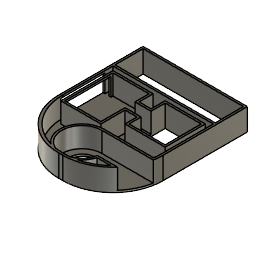
[vacc]base2 (Autodesk Fusion 360 design; units mm, degrees)
part number: 2026-07-20-20-28-10-473
Autodesk Fusion 360 part; units mm, degrees
sketch "Sketch1" plane through (0, 0, 0) normal (0, 0, 1) x (1, 0, 0)
  line L0 (-25, 25) -> (235, 25)
  line L1 (235, 25) -> (235, -110)
  line L2 (110, -235) -> (100, -235)
  line L3 (-25, -110) -> (-25, 25)
  line L4 (-25, 25) -> (-20, 25)
  line L5 (-20, 25) -> (-20, 20)
  line L6 (-20, 20) -> (-25, 20)
  line L7 (-25, 20) -> (-25, 25)
  line L8 (235, 25) -> (230, 25)
  line L9 (230, 25) -> (230, 20)
  line L10 (230, 20) -> (235, 20)
  line L11 (235, 20) -> (235, 25)
  line L12 (-25, -235) -> (-20, -235)
  line L13 (-20, -235) -> (-20, -230)
  line L14 (-20, -230) -> (-25, -230)
  line L15 (-25, -230) -> (-25, -235)
  line L16 (235, -235) -> (230, -235)
  line L17 (230, -235) -> (230, -230)
  line L18 (230, -230) -> (235, -230)
  line L19 (235, -230) -> (235, -235)
  line L20 (-20, 20) -> (230, 20)
  line L21 (230, 20) -> (230, -110)
  line L22 (110, -230) -> (100, -230)
  line L23 (-20, -110) -> (-20, 20)
  arc A0 (-20, -110) -> (100, -230) centre (100, -110) ccw
  arc A1 (-25, -110) -> (100, -235) centre (100, -110) ccw
  arc A2 (110, -230) -> (230, -110) centre (110, -110) ccw
  arc A3 (110, -235) -> (235, -110) centre (110, -110) ccw
  dimension "d1" = 260
  dimension "d2" = 260
  dimension "d3" = 5
  dimension "d4" = 5
  dimension "d5" = 120
  dimension "d6" = 125
  dimension "d7" = 120
  dimension "d8" = 125
  constraint horizontal L0
  constraint vertical L1
  constraint horizontal L2
  constraint vertical L3
  constraint horizontal L4
  constraint vertical L5
  constraint horizontal L6
  constraint vertical L7
  constraint horizontal L8
  constraint vertical L9
  constraint horizontal L10
  constraint vertical L11
  constraint horizontal L12
  constraint vertical L13
  constraint horizontal L14
  constraint vertical L15
  constraint horizontal L16
  constraint vertical L17
  constraint horizontal L18
  constraint vertical L19
  constraint horizontal L20
  constraint vertical L21
  constraint horizontal L22
  constraint vertical L23
  constraint tangent L23 A0
  constraint tangent L22 A0
  constraint coincident L12.start L3
  constraint coincident L12.start L2
  constraint tangent L3 A1
  constraint tangent L2 A1
  constraint coincident L17.end L21
  constraint coincident L17.end L22
  constraint tangent L21 A2
  constraint tangent L22 A2
  constraint coincident L16.start L2
  constraint coincident L16.start L1
  constraint tangent L2 A3
  constraint tangent L1 A3
  measures "d1" distance of L0.start L12.start
  measures "d2" distance of L0.start L0.end
  measures "d3" distance of L0.start L4.end
  measures "d4" distance of L0.start L6.end
  measures "d5" radius of A0
  measures "d6" radius of A1
  measures "d7" radius of A2
  measures "d8" radius of A3
extrude "Extrude1" add sketch "Sketch1" along normal blind 5 contours L0 L3 L4 L5 L6 L7 | L0 L5 L9 L20 | L1 L2 L3 L6 L10 L21 L22 L23 A0 A1 A2 A3 | L0 L1 L8 L9 L10 L11 | L20 L21 L22 L23 A0 A2
sketch "Sketch2" plane through (0, 0, 5) normal (0, 0, 1) x (-1, 0, 0)
  arc A0 (25, 110) -> (-100, 235) centre (-100, 110) ccw
  line L0 (-100, 235) -> (-110, 235)
  arc A1 (-110, 235) -> (-235, 110) centre (-110, 110) ccw
  line L1 (-235, 110) -> (-235, -25)
  line L2 (-235, -25) -> (25, -25)
  line L3 (25, -25) -> (25, 110)
  line L4 (25, -25) -> (-235, -25)
  line L5 (-235, -25) -> (-235, 110)
  line L6 (-110, 235) -> (-100, 235)
  line L7 (25, 110) -> (25, -25)
  line L8 (25, -25) -> (20, -25)
  line L9 (20, -25) -> (20, -20)
  line L10 (20, -20) -> (25, -20)
  line L11 (25, -20) -> (25, -25)
  line L12 (-235, -25) -> (-230, -25)
  line L13 (-230, -25) -> (-230, -20)
  line L14 (-230, -20) -> (-235, -20)
  line L15 (-235, -20) -> (-235, -25)
  line L16 (25, 235) -> (20, 235)
  line L17 (20, 235) -> (20, 230)
  line L18 (20, 230) -> (25, 230)
  line L19 (25, 230) -> (25, 235)
  line L20 (-235, 235) -> (-230, 235)
  line L21 (-230, 235) -> (-230, 230)
  line L22 (-230, 230) -> (-235, 230)
  line L23 (-235, 230) -> (-235, 235)
  line L24 (20, -20) -> (-230, -20)
  line L25 (-230, -20) -> (-230, 110)
  line L26 (-110, 230) -> (-105, 230)
  line L27 (20, 105) -> (20, -20)
  arc A2 (20, 105) -> (-105, 230) centre (-105, 105) ccw
  arc A3 (25, 110) -> (-100, 235) centre (-100, 110) ccw
  arc A4 (-110, 230) -> (-230, 110) centre (-110, 110) ccw
  arc A5 (-110, 235) -> (-235, 110) centre (-110, 110) ccw
  dimension "d11" = 260
  dimension "d12" = 260
  dimension "d13" = 5
  dimension "d14" = 5
  dimension "d15" = 5
  dimension "d16" = 5
  dimension "d17" = 125
  dimension "d18" = 120
  dimension "d19" = 125
  constraint horizontal L4
  constraint vertical L5
  constraint horizontal L6
  constraint vertical L7
  constraint coincident L2.end L3.start
  constraint horizontal L8
  constraint vertical L9
  constraint horizontal L10
  constraint vertical L11
  constraint horizontal L12
  constraint vertical L13
  constraint horizontal L14
  constraint vertical L15
  constraint coincident L1.end L2.start
  constraint horizontal L16
  constraint vertical L17
  constraint horizontal L18
  constraint vertical L19
  constraint horizontal L20
  constraint vertical L21
  constraint horizontal L22
  constraint vertical L23
  constraint horizontal L24
  constraint vertical L25
  constraint horizontal L26
  constraint vertical L27
  constraint tangent L27 A2
  constraint tangent L26 A2
  constraint coincident L16.start L7
  constraint coincident L16.start L6
  constraint tangent L7 A3
  constraint tangent L6 A3
  constraint equal A2 A3
  constraint coincident L21.end L25
  constraint coincident L21.end L26
  constraint tangent L25 A4
  constraint tangent L26 A4
  constraint coincident L20.start L6
  constraint coincident L20.start L5
  constraint tangent L6 A5
  constraint tangent L5 A5
  measures "d11" distance of L2.end L16.start
  measures "d12" distance of L20.start L16.start
  measures "d13" distance of L17.end L18.end
  measures "d14" distance of L16.end L17.end
  measures "d15" distance of L21.end L22.end
  measures "d16" distance of L20.end L21.end
  measures "d17" radius of A2
  measures "d18" radius of A4
  measures "d19" radius of A5
extrude "Extrude2" add sketch "Sketch2" along normal blind 50 contours A0 L0 A1 L1 L3 L5 L6 L7 L10 L14 L25 L26 L27 A2 A3 A4 A5 | L2 L3 L4 L7 L8 L9 L10 L11 | L2 L4 L9 L13 L24 | L1 L2 L4 L5 L12 L13 L14 L15
sketch "Sketch3" plane through (0, 0, 5) normal (0, 0, 1) x (-1, 0, 0)
  line L0 (-105, 230) -> (-110, 230)
  arc A0 (-110, 230) -> (-230, 110) centre (-110, 110) ccw
  line L1 (-230, 110) -> (-230, -20)
  line L2 (-230, -20) -> (20, -20)
  line L3 (20, -20) -> (20, 105)
  arc A1 (20, 105) -> (-105, 230) centre (-105, 105) ccw
  line L4 (-230, -20) -> (-220, -20)
  line L5 (-220, -20) -> (-220, -10)
  line L6 (-220, -10) -> (-120, -10)
  line L7 (-120, -10) -> (-120, 90)
  line L8 (-120, 90) -> (-220, 90)
  line L9 (-220, 90) -> (-220, -10)
  line L10 (20, -20) -> (20, -10)
  line L11 (20, -20) -> (10, -20)
  line L12 (20, -20) -> (10, -20)
  line L13 (10, -20) -> (10, -10)
  line L14 (10, -10) -> (20, -10)
  line L15 (20, -10) -> (20, -20)
  line L16 (10, -10) -> (-90, -10)
  line L17 (-90, -10) -> (-90, 120)
  line L18 (-90, 120) -> (10, 120)
  line L19 (10, 120) -> (10, -10)
  line L20 (-90, -10) -> (-90, 30)
  line L21 (-120, -10) -> (-120, 30)
  line L22 (-120, 30) -> (-90, 30)
  line L23 (-90, 30) -> (-90, 55)
  line L24 (-90, 55) -> (-120, 55)
  line L25 (-120, 55) -> (-120, 30)
  line L26 (10, -10) -> (5, -10)
  line L27 (5, -10) -> (5, -5)
  line L28 (5, -5) -> (10, -5)
  line L29 (10, -5) -> (10, -10)
  line L30 (-90, -10) -> (-85, -10)
  line L31 (-85, -10) -> (-85, -5)
  line L32 (-85, -5) -> (-90, -5)
  line L33 (-90, -5) -> (-90, -10)
  line L34 (10, 120) -> (5, 120)
  line L35 (5, 120) -> (5, 115)
  line L36 (5, 115) -> (10, 115)
  line L37 (10, 115) -> (10, 120)
  line L38 (-90, 120) -> (-85, 120)
  line L39 (-85, 120) -> (-85, 115)
  line L40 (-85, 115) -> (-90, 115)
  line L41 (-90, 115) -> (-90, 120)
  line L42 (5, -5) -> (-85, -5)
  line L43 (-85, -5) -> (-85, 115)
  line L44 (-85, 115) -> (5, 115)
  line L45 (5, 115) -> (5, -5)
  line L46 (-90, 30) -> (-90, 25)
  line L47 (-120, 30) -> (-120, 25)
  line L48 (-120, 25) -> (-90, 25)
  line L49 (-90, 55) -> (-90, 60)
  line L50 (-120, 55) -> (-120, 60)
  line L51 (-120, 60) -> (-90, 60)
  line L52 (-120, -10) -> (-125, -10)
  line L53 (-125, -10) -> (-125, -5)
  line L54 (-125, -5) -> (-120, -5)
  line L55 (-120, -5) -> (-120, -10)
  line L56 (-220, -10) -> (-215, -10)
  line L57 (-215, -10) -> (-215, -5)
  line L58 (-215, -5) -> (-220, -5)
  line L59 (-220, -5) -> (-220, -10)
  line L60 (-120, 90) -> (-125, 90)
  line L61 (-125, 90) -> (-125, 85)
  line L62 (-125, 85) -> (-120, 85)
  line L63 (-120, 85) -> (-120, 90)
  line L64 (-220, 90) -> (-215, 90)
  line L65 (-215, 90) -> (-215, 85)
  line L66 (-215, 85) -> (-220, 85)
  line L67 (-220, 85) -> (-220, 90)
  line L68 (-125, -5) -> (-215, -5)
  line L69 (-215, -5) -> (-215, 85)
  line L70 (-215, 85) -> (-125, 85)
  line L71 (-125, 85) -> (-125, -5)
  dimension "d22" = 10
  dimension "d23" = 10
  dimension "d24" = 100
  dimension "d25" = 100
  dimension "d26" = 10
  dimension "d27" = 10
  dimension "d28" = 100
  dimension "d29" = 130
  dimension "d30" = 40
  dimension "d31" = 30
  dimension "d32" = 25
  dimension "d33" = 5
  dimension "d34" = 5
  constraint coincident L1.end L2.start
  constraint perpendicular L1 L4
  constraint perpendicular L4 L5
  constraint horizontal L6
  constraint vertical L7
  constraint horizontal L8
  constraint vertical L9
  constraint coincident L2.end L3.start
  constraint perpendicular L2 L10
  constraint coincident L2 L11.end
  constraint horizontal L12
  constraint vertical L13
  constraint horizontal L14
  constraint vertical L15
  constraint horizontal L16
  constraint vertical L17
  constraint horizontal L18
  constraint vertical L19
  constraint coincident L17 L20.end
  constraint perpendicular L16 L21
  constraint horizontal L22
  constraint vertical L23
  constraint horizontal L24
  constraint vertical L25
  constraint midpoint L17 L23.end
  constraint horizontal L26
  constraint vertical L27
  constraint horizontal L28
  constraint vertical L29
  constraint horizontal L30
  constraint vertical L31
  constraint horizontal L32
  constraint vertical L33
  constraint horizontal L34
  constraint vertical L35
  constraint horizontal L36
  constraint vertical L37
  constraint horizontal L38
  constraint vertical L39
  constraint horizontal L40
  constraint vertical L41
  constraint horizontal L42
  constraint vertical L43
  constraint horizontal L44
  constraint vertical L45
  constraint coincident L17 L46.end
  constraint coincident L21 L47.end
  constraint perpendicular L46 L48
  constraint coincident L17 L49.end
  constraint coincident L7 L50.end
  constraint perpendicular L49 L51
  constraint horizontal L52
  constraint vertical L53
  constraint horizontal L54
  constraint vertical L55
  constraint horizontal L56
  constraint vertical L57
  constraint horizontal L58
  constraint vertical L59
  constraint horizontal L60
  constraint vertical L61
  constraint horizontal L62
  constraint vertical L63
  constraint horizontal L64
  constraint vertical L65
  constraint horizontal L66
  constraint vertical L67
  constraint horizontal L68
  constraint vertical L69
  constraint horizontal L70
  constraint vertical L71
  measures "d22" distance of L1.end L4.end
  measures "d23" distance of L4.end L5.end
  measures "d24" distance of L5.end L6.end
  measures "d25" distance of L5.end L8.end
  measures "d26" distance of L1 L8.end
  measures "d27" distance of L2.end L10.end
  measures "d28" distance of L13.end L16.end
  measures "d29" distance of L13.end L18.end
  measures "d30" distance of L6.end L21.end
  measures "d31" distance of L21.end L20.end
  measures "d32" distance of L20.end L23.end
  measures "d33" distance of L21.end L47.end
  measures "d34" distance of L24.end L50.end
extrude "Extrude3" add sketch "Sketch3" along normal blind 50 contours L16 L19 L26 L27 L28 L29 | L16 L27 L31 L42 | L19 L28 L36 L45 | L6 L9 L56 L57 L58 L59 | L16 L17 L20 L30 L31 L32 L33 | L18 L19 L34 L35 L36 L37 | L6 L53 L57 L68 | L9 L58 L66 L69 | L17 L20 L23 L32 L40 L43 L46 L49 | L18 L35 L39 L44 | L6 L7 L21 L52 L53 L54 L55 | L8 L9 L64 L65 L66 L67 | L17 L18 L38 L39 L40 L41 | L7 L21 L25 L47 L50 L54 L62 L71 | L8 L61 L65 L70 | L7 L17 L20 L21 L22 L46 L47 L48 | L7 L8 L60 L61 L62 L63 | L7 L17 L24 L49 L50 L51
extrude "Extrude4" cut 1 faces at (90, -38.3333, 21.6667) along direction (-1, 0, 0) blind 20
extrude "Extrude5" cut 1 faces at (120, -38.3333, 21.6667) along direction (1, 0, 0) blind 30
sketch "Sketch4" plane through (0, 0, 5) normal (0, 0, 1) x (-1, 0, 0)
  line L0 (-85, 55) -> (-125, 55)
  line L1 (-125, 55) -> (-125, 85)
  line L2 (-125, 85) -> (-215, 85)
  line L3 (-215, 85) -> (-215, -5)
  line L4 (-215, -5) -> (-125, -5)
  line L5 (-125, -5) -> (-125, 30)
  line L6 (-125, 30) -> (-85, 30)
  line L7 (-85, 30) -> (-85, -5)
  line L8 (-85, -5) -> (5, -5)
  line L9 (5, -5) -> (5, 115)
  line L10 (5, 115) -> (-85, 115)
  line L11 (-85, 115) -> (-85, 55)
  line L12 (-125, -5) -> (-215, -5)
  line L13 (-215, -5) -> (-215, 85)
  line L14 (-215, 85) -> (-125, 85)
  line L15 (-125, 85) -> (-125, -5)
  constraint horizontal L12
  constraint vertical L13
  constraint horizontal L14
  constraint vertical L15
  constraint coincident L2.end L3.start
  constraint coincident L4.end L5.start
extrude "Extrude6" cut sketch "Sketch4" against normal blind 30 contours L1 L2 L3 L4 L5 L12 L13 L14 L15
sketch "Sketch5" plane through (0, 0, 5) normal (0, 0, 1) x (-1, 0, 0)
  line L0 (-105, 230) -> (-110, 230)
  arc A0 (-110, 230) -> (-230, 110) centre (-110, 110) ccw
  line L1 (-230, 110) -> (-230, -20)
  line L2 (-230, -20) -> (20, -20)
  line L3 (20, -20) -> (20, 105)
  arc A1 (20, 105) -> (-105, 230) centre (-105, 105) ccw
  line L4 (-220, 90) -> (-120, 90)
  line L5 (-120, 90) -> (-120, 60)
  line L6 (-120, 60) -> (-90, 60)
  line L7 (-90, 60) -> (-90, 120)
  line L8 (-90, 120) -> (10, 120)
  line L9 (10, 120) -> (10, -10)
  line L10 (10, -10) -> (-90, -10)
  line L11 (-90, -10) -> (-90, 25)
  line L12 (-90, 25) -> (-120, 25)
  line L13 (-120, 25) -> (-120, -10)
  line L14 (-120, -10) -> (-220, -10)
  line L15 (-220, -10) -> (-220, 90)
  line L16 (25, -25) -> (-235, -25)
  line L17 (-235, -25) -> (-235, 235)
  line L18 (-235, 235) -> (25, 235)
  line L19 (25, 235) -> (25, -25)
  line L20 (25, -25) -> (20, -25)
  line L21 (20, -25) -> (20, -20)
  line L22 (20, -20) -> (25, -20)
  line L23 (25, -20) -> (25, -25)
  line L24 (-235, -25) -> (-230, -25)
  line L25 (-230, -25) -> (-230, -20)
  line L26 (-230, -20) -> (-235, -20)
  line L27 (-235, -20) -> (-235, -25)
  line L28 (25, 235) -> (20, 235)
  line L29 (20, 235) -> (20, 230)
  line L30 (20, 230) -> (25, 230)
  line L31 (25, 230) -> (25, 235)
  line L32 (-235, 235) -> (-230, 235)
  line L33 (-230, 235) -> (-230, 232.5)
  line L34 (-230, 232.5) -> (-235, 232.5)
  line L35 (-235, 232.5) -> (-235, 235)
  line L36 (20, -20) -> (-230, -20)
  line L37 (-230, -20) -> (-230, 232.5)
  line L38 (-230, 232.5) -> (20, 232.5)
  line L39 (20, 232.5) -> (20, -20)
  line L40 (20, 232.5) -> (20, 182.5)
  line L41 (-230, 232.5) -> (-230, 182.5)
  line L42 (20, 182.5) -> (-105, 182.5)
  circle A2 centre (-105, 182.5) radius 50
  line L43 (-55, 182.5) -> (-155, 182.5)
  line L44 (-155, 182.5) -> (-155, 235)
  line L45 (-155, 235) -> (-55, 235)
  line L46 (-55, 235) -> (-55, 182.5)
  line L47 (-230, 182.5) -> (-230, 142.5)
  line L48 (-105, 182.5) -> (-105, 132.5)
  line L49 (-105, 132.5) -> (-235, 132.5)
  line L50 (-230, 132.5) -> (-230, 182.5)
  line L51 (-230, 182.5) -> (-230, 192.5)
  line L52 (-230, 192.5) -> (-153.9898, 192.5)
  circle A3 centre (-105, 182.5) radius 55
  line L53 (-105, 127.5) -> (-235, 127.5)
  line L54 (-230, 192.5) -> (-230, 197.5)
  line L55 (-230, 132.5) -> (-230, 192.5)
  line L56 (20, 182.5) -> (-160, 182.5)
  line L57 (-230, 197.5) -> (-157.915, 197.5)
  dimension "d43" = 260
  dimension "d44" = 260
  dimension "d45" = 5
  dimension "d46" = 5
  dimension "d47" = 50
  dimension "d48" = 50
  dimension "d49" = 125
  dimension "d50" = 100
  dimension "d51" = 40
  dimension "d52" = 50
  dimension "d53" = 10
  dimension "d54" = 110
  dimension "d55" = 5
  dimension "d56" = 5
  dimension "d57" = 60
  constraint horizontal L16
  constraint vertical L17
  constraint horizontal L18
  constraint vertical L19
  constraint horizontal L20
  constraint vertical L21
  constraint horizontal L22
  constraint vertical L23
  constraint coincident L2.end L3.start
  constraint horizontal L24
  constraint vertical L25
  constraint horizontal L26
  constraint vertical L27
  constraint coincident L1.end L2.start
  constraint horizontal L28
  constraint vertical L29
  constraint horizontal L30
  constraint vertical L31
  constraint horizontal L32
  constraint vertical L33
  constraint horizontal L34
  constraint vertical L35
  constraint horizontal L36
  constraint vertical L37
  constraint horizontal L38
  constraint vertical L39
  constraint perpendicular L38 L40
  constraint perpendicular L38 L41
  constraint coincident L42.end A2.centre
  constraint horizontal L43
  constraint vertical L44
  constraint horizontal L45
  constraint vertical L46
  constraint coincident L18 L44.end
  constraint coincident A2 L43.start
  constraint coincident L43.start L56
  constraint coincident A2 L48.end
  constraint perpendicular L42 L48
  constraint coincident L17 L49.end
  constraint perpendicular L17 L49
  constraint coincident L49 L50.start
  constraint coincident L37 L50.start
  constraint coincident A2 L52.end
  constraint perpendicular L44 L52
  constraint concentric A2 A3
  constraint coincident A3 L53.start
  constraint coincident L17 L53.end
  constraint tangent A3 L53
  constraint perpendicular L17 L53
  constraint perpendicular L52 L54
  constraint parallel L41 L55
  constraint coincident A3 L56.end
  constraint coincident L42.end L56
  constraint coincident A3 L57.end
  constraint perpendicular L54 L57
  measures "d43" distance of L16.start L16.end
  measures "d44" distance of L16.start L18.end
  measures "d45" distance of L29.end L30.end
  measures "d46" distance of L28.end L29.end
  measures "d47" distance of L38.end L40.end
  measures "d48" distance of L33.end L41.end
  measures "d49" distance of L40.end L42.end
  measures "d50" diameter of A2
  measures "d51" distance of L41.end L47.end
  measures "d52" distance of L41.end L50.start
  measures "d53" distance of L41.end L51.end
  measures "d54" diameter of A3
  measures "d55" distance of L51.end L54.end
  measures "d56" distance of L49 L53
  measures "d57" distance of L50.start L51.end
extrude "Extrude7" add sketch "Sketch5" along normal blind 50 contours A1 A2 L46 A3 | A0 A2 L44 L52 A3 | L42 L46 A3 L56 | L42 A2 L49 A3 L56 | L44 L52 A3 | A0 L49 A3 L53 | A0 L52 A3 L57
sketch "Sketch6" plane through (0, 0, 5) normal (0, 0, 1) x (-1, 0, 0)
  line L0 (-227.8718, 132.5) -> (-105, 132.5)
  arc A0 (-105, 132.5) -> (-85.2346, 228.4274) centre (-105, 182.5) ccw
  arc A1 (-85.2346, 228.4274) -> (-105, 230) centre (-105, 105) ccw
  line L1 (-105, 230) -> (-110, 230)
  arc A2 (-110, 230) -> (-122.4639, 229.351) centre (-110, 110) ccw
  arc A3 (-122.4639, 229.351) -> (-153.9898, 192.5) centre (-105, 182.5) ccw
  line L2 (-153.9898, 192.5) -> (-197.1421, 192.5)
  arc A4 (-197.1421, 192.5) -> (-227.8718, 132.5) centre (-110, 110) ccw
  line L3 (25.0024, -24.9997) -> (-234.9976, -24.9997)
  line L4 (-234.9976, -24.9997) -> (-234.9976, 235.0003)
  line L5 (-234.9976, 235.0003) -> (25.0024, 235.0003)
  line L6 (25.0024, 235.0003) -> (25.0024, -24.9997)
  line L7 (25.0024, -24.9997) -> (20.0024, -24.9997)
  line L8 (20.0024, -24.9997) -> (20.0024, -19.9997)
  line L9 (20.0024, -19.9997) -> (25.0024, -19.9997)
  line L10 (25.0024, -19.9997) -> (25.0024, -24.9997)
  line L11 (-234.9976, -24.9997) -> (-229.9976, -24.9997)
  line L12 (-229.9976, -24.9997) -> (-229.9976, -20)
  line L13 (-229.9976, -20) -> (-234.9976, -20)
  line L14 (-234.9976, -20) -> (-234.9976, -24.9997)
  line L15 (25.0024, 235.0003) -> (20.0024, 235.0003)
  line L16 (20.0024, 235.0003) -> (20.0024, 230)
  line L17 (20.0024, 230) -> (25.0024, 230)
  line L18 (25.0024, 230) -> (25.0024, 235.0003)
  line L19 (-234.9976, 235.0003) -> (-229.9976, 235.0003)
  line L20 (-229.9976, 235.0003) -> (-229.9976, 230)
  line L21 (-229.9976, 230) -> (-234.9976, 230)
  line L22 (-234.9976, 230) -> (-234.9976, 235.0003)
  line L23 (20.0024, -19.9997) -> (-229.9976, -19.9997)
  line L24 (-229.9976, -19.9997) -> (-229.9976, 230)
  line L25 (-229.9976, 230) -> (20.0024, 230)
  line L26 (20.0024, 230) -> (20.0024, -19.9997)
  line L27 (20.0024, 230) -> (20.0024, 180)
  line L28 (-229.9976, 230) -> (-229.9976, 180)
  line L29 (20.0024, 180) -> (-229.9976, 180)
  line L30 (20.0024, 180) -> (-104.9976, 180)
  circle A5 centre (-104.9976, 180) radius 32
  dimension "d60" = 260
  dimension "d61" = 260
  dimension "d62" = 5
  dimension "d63" = 5
  dimension "d64" = 5
  dimension "d65" = 5
  dimension "d66" = 5
  dimension "d67" = 50
  dimension "d68" = 50
  dimension "d69" = 125
  dimension "d70" = 64
  constraint horizontal L3
  constraint vertical L4
  constraint horizontal L5
  constraint vertical L6
  constraint horizontal L7
  constraint vertical L8
  constraint horizontal L9
  constraint vertical L10
  constraint horizontal L11
  constraint vertical L12
  constraint horizontal L13
  constraint vertical L14
  constraint horizontal L15
  constraint vertical L16
  constraint horizontal L17
  constraint vertical L18
  constraint horizontal L19
  constraint vertical L20
  constraint horizontal L21
  constraint vertical L22
  constraint horizontal L23
  constraint vertical L24
  constraint horizontal L25
  constraint vertical L26
  constraint perpendicular L17 L27
  constraint perpendicular L25 L28
  constraint perpendicular L24 L29
  constraint midpoint L29 L30.end
  constraint coincident L30.end A5.centre
  measures "d60" distance of L3.start L5.end
  measures "d61" distance of L4.end L5.end
  measures "d62" distance of L3.start L9.end
  measures "d63" distance of L3.start L7.end
  measures "d64" distance of L3.end L11.end
  measures "d65" distance of L5.end L15.end
  measures "d66" distance of L4.end L19.end
  measures "d67" distance of L16.end L27.end
  measures "d68" distance of L20.end L28.end
  measures "d69" distance of L27.end L30.end
  measures "d70" diameter of A5
extrude "Extrude8" cut sketch "Sketch6" against normal blind 30 contours L29 L30 A5 | L29 L30 A5
sketch "Sketch7" plane through (0, 0, 5) normal (0, 0, 1) x (-1, 0, 0)
  circle A0 centre (-104.9976, 180) radius 32
  line L0 (-227.8718, 132.5) -> (-105, 132.5)
  arc A1 (-105, 132.5) -> (-85.2346, 228.4274) centre (-105, 182.5) ccw
  arc A2 (-85.2346, 228.4274) -> (-105, 230) centre (-105, 105) ccw
  line L1 (-105, 230) -> (-110, 230)
  arc A3 (-110, 230) -> (-122.4639, 229.351) centre (-110, 110) ccw
  arc A4 (-122.4639, 229.351) -> (-153.9898, 192.5) centre (-105, 182.5) ccw
  line L2 (-153.9898, 192.5) -> (-197.1421, 192.5)
  arc A5 (-197.1421, 192.5) -> (-227.8718, 132.5) centre (-110, 110) ccw
  line L3 (-180.0058, 132.5) -> (-234.0378, 132.5)
  line L4 (-234.0378, 132.5) -> (-234.0378, 192.5014)
  line L5 (-234.0378, 192.5014) -> (-180.0058, 192.5014)
  line L6 (-180.0058, 192.5014) -> (-180.0058, 132.5)
  constraint horizontal L3
  constraint vertical L4
  constraint horizontal L5
  constraint vertical L6
  constraint coincident L0 L3.start
extrude "Extrude9" cut sketch "Sketch7" along normal blind 60 contours L2 A5 L3 L4 L5 L6
sketch "Sketch8" plane through (0, 0, 5) normal (0, 0, 1) x (-1, 0, 0)
  line L0 (-125, 55) -> (-125, 30)
  line L1 (-125, 30) -> (-85, 30)
  line L2 (-85, 30) -> (-85, -5)
  line L3 (-85, -5) -> (5, -5)
  line L4 (5, -5) -> (5, 115)
  line L5 (5, 115) -> (-85, 115)
  line L6 (-85, 115) -> (-85, 55)
  line L7 (-85, 55) -> (-125, 55)
  line L8 (25, -25) -> (-235, -25)
  line L9 (-235, -25) -> (-235, -100)
  line L10 (-235, -100) -> (25, -100)
  line L11 (25, -100) -> (25, -25)
  line L12 (25, -100) -> (20, -100)
  line L13 (20, -100) -> (20, -95)
  line L14 (20, -95) -> (25, -95)
  line L15 (25, -95) -> (25, -100)
  line L16 (-235, -100) -> (-230, -100)
  line L17 (-230, -100) -> (-230, -95)
  line L18 (-230, -95) -> (-235, -95)
  line L19 (-235, -95) -> (-235, -100)
  line L20 (25, -25) -> (20, -25)
  line L21 (20, -25) -> (20, -20)
  line L22 (20, -20) -> (25, -20)
  line L23 (25, -20) -> (25, -25)
  line L24 (-235, -25) -> (-230, -25)
  line L25 (-230, -25) -> (-230, -20)
  line L26 (-230, -20) -> (-235, -20)
  line L27 (-235, -20) -> (-235, -25)
  line L28 (20, -95) -> (-230, -95)
  line L29 (-230, -95) -> (-230, -25)
  line L30 (-230, -25) -> (20, -25)
  line L31 (20, -25) -> (20, -95)
  dimension "d75" = 75
  constraint horizontal L8
  constraint vertical L9
  constraint horizontal L10
  constraint vertical L11
  constraint horizontal L12
  constraint vertical L13
  constraint horizontal L14
  constraint vertical L15
  constraint horizontal L16
  constraint vertical L17
  constraint horizontal L18
  constraint vertical L19
  constraint horizontal L20
  constraint vertical L21
  constraint horizontal L22
  constraint vertical L23
  constraint horizontal L24
  constraint vertical L25
  constraint horizontal L26
  constraint vertical L27
  constraint horizontal L28
  constraint vertical L29
  constraint horizontal L30
  constraint vertical L31
  measures "d75" distance of L8.start L10.end
extrude "Extrude10" add sketch "Sketch8" along normal blind 50 contours L8 L11 L14 L20 L31 | L10 L11 L12 L13 L14 L15 | L8 L9 L18 L24 L29 | L10 L13 L17 L28 | L9 L10 L16 L17 L18 L19
extrude "Extrude11" add 1 faces at (63.3333, 98.3333, 5) along direction (0, 0, -1) blind 5
sketch "Sketch9" plane through (-5, 0, 0) normal (1, 0, 0) x (0, 1, 0)
  line L0 (-115, 5) -> (5, 5)
  line L1 (5, 5) -> (5, 55)
  line L2 (5, 55) -> (-115, 55)
  line L3 (-115, 55) -> (-115, 5)
  line L4 (5, 5) -> (-115, 5)
  line L5 (-115, 5) -> (-115, 0)
  line L6 (-115, 0) -> (5, 0)
  line L7 (5, 0) -> (5, 5)
  line L8 (0, 5) -> (-110, 5)
  line L9 (-110, 5) -> (-110, 50)
  line L10 (-110, 50) -> (0, 50)
  line L11 (0, 50) -> (0, 5)
  constraint horizontal L4
  constraint vertical L5
  constraint horizontal L6
  constraint vertical L7
  constraint coincident L0.end L1.start
  constraint horizontal L8
  constraint vertical L9
  constraint horizontal L10
  constraint vertical L11
  constraint coincident L4 L8.start
extrude "Extrude12" cut sketch "Sketch9" against normal blind 70 contours L0 L4 L8 L9 L10 L11
